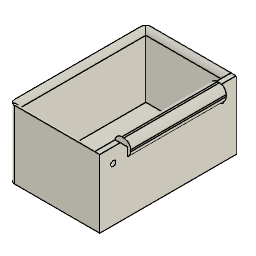
Caja Receptora Lateral (Autodesk Fusion 360 design; units mm, degrees)
Autodesk Fusion 360 part; units mm, degrees
sketch "Boceto1" plane through (0, 0, 0) normal (1, 0, 0) x (0, 1, 0)
  line L0 (0, 0) -> (80, 0)
  line L1 (80, 0) -> (80, 40)
  line L2 (80, 40) -> (0, 40)
  line L3 (0, 40) -> (0, 0)
  line L4 (80, 40) -> (80, 33)
  line L5 (80, 33) -> (80, 31.5)
  line L6 (80, 31.5) -> (72.1, 31.5)
  line L7 (0, 40) -> (0, 38.7984)
  line L8 (0, 40) -> (0, 33)
  line L9 (0, 33) -> (0, 31.5)
  line L10 (0, 31.5) -> (7.9, 31.5)
  circle A0 centre (7.9, 31.5) radius 1.525
  circle A1 centre (72.1, 31.5) radius 1.525
  dimension "d1" = 80
  dimension "d2" = 40
  dimension "d3" = 7
  dimension "d4" = 1.5
  dimension "d5" = 7.9
  dimension "d6" = 7
  dimension "d7" = 1.5
  dimension "d8" = 7.9
  dimension "d9" = 3.05
  dimension "d10" = 3.05
  constraint horizontal L0
  constraint vertical L1
  constraint horizontal L2
  constraint vertical L3
  constraint coincident L0.start L3.end
  constraint perpendicular L2 L4
  constraint perpendicular L2 L5
  constraint perpendicular L1 L6
  constraint coincident L3 L7.end
  constraint perpendicular L2 L8
  constraint perpendicular L2 L9
  constraint perpendicular L3 L10
  constraint coincident L10.end A0.centre
  constraint coincident L6.end A1.centre
  measures "d1" distance of L0.start L0.end
  measures "d2" distance of L0.start L2.end
  measures "d3" distance of L1.end L4.end
  measures "d4" distance of L4.end L5.end
  measures "d5" distance of L5.end L6.end
  measures "d6" distance of L2.end L8.end
  measures "d7" distance of L8.end L9.end
  measures "d8" distance of L9.end L10.end
  measures "d9" diameter of A0
  measures "d10" diameter of A1
extrude "Extruir1" add sketch "Boceto1" against normal blind 2 makes body 1
sketch "Boceto2" plane through (-2, 0, 0) normal (-1, 0, 0) x (0, -1, 0)
  circle A0 centre (-7.9, 31.5) radius 1.525
  circle A1 centre (-72.1, 31.5) radius 1.525
  line L0 (0, 40) -> (-80, 40)
  line L1 (-80, 40) -> (-80, 0)
  line L2 (-80, 0) -> (0, 0)
  line L3 (0, 0) -> (0, 40)
extrude "Extruir2" add sketch "Boceto2" along normal blind 1 contours A0 | A1 | L0 L1 L2 L3 bodies 1
sketch "Boceto3" plane through (0, 0, 40) normal (0, 0, 1) x (-1, 0, 0)
  line L0 (0, 0) -> (0, -80)
  line L1 (0, -80) -> (3, -80)
  line L2 (3, -80) -> (3, 0)
  line L3 (3, 0) -> (0, 0)
  line L4 (3, -80) -> (53, -80)
  line L5 (53, -80) -> (53, 0)
  line L6 (53, 0) -> (3, 0)
  line L7 (3, 0) -> (3, -80)
  line L8 (50, -3) -> (6, -3)
  line L9 (6, -3) -> (6, -77)
  line L10 (6, -77) -> (50, -77)
  line L11 (50, -77) -> (50, -3)
  line L12 (6, -77) -> (3, -77)
  line L13 (6, -3) -> (3, -3)
  dimension "d15" = 50
  dimension "d16" = -3
  constraint horizontal L4
  constraint vertical L5
  constraint horizontal L6
  constraint vertical L7
  constraint coincident L1.end L2.start
  constraint coincident L7 L12.end
  constraint perpendicular L7 L12
  constraint coincident L7 L13.end
  constraint perpendicular L7 L13
  constraint coincident L2.end L3.start
  measures "d15" distance of L1.end L4.end
extrude "Extruir3" add sketch "Boceto3" against normal up to surface (40 mm away) contours L2 L4 L5 L6 L7 L8 L10 L11 L12 L13 bodies 1
sketch "Boceto4" plane through (0, 0, 0) normal (0, 0, -1) x (1, 0, 0)
  line L0 (-3, -3) -> (-3, -77)
  line L1 (-3, -77) -> (-50, -77)
  line L2 (-50, -77) -> (-50, -3)
  line L3 (-50, -3) -> (-3, -3)
  line L4 (0, 0) -> (-53, 0)
  line L5 (-53, 0) -> (-53, -80)
  line L6 (-53, -80) -> (0, -80)
  line L7 (0, -80) -> (0, 0)
extrude "Extruir4" add sketch "Boceto4" against normal blind 3 contours L0 L1 L2 L3 bodies 1
copy_body "Cuerpo - > Comp.1" bodies 1 removing the originals makes body 2 in component "Caja Receptora"
sketch "Boceto5" plane through (0, 0, 0) normal (0, -1, 0) x (1, 0, 0)
  line L0 (0, 0) -> (0, 40)
  line L1 (0, 40) -> (-53, 40)
  line L2 (-53, 40) -> (-53, 0)
  line L3 (-53, 0) -> (0, 0)
  line L4 (0, 40) -> (-3, 40)
  line L5 (-3, 40) -> (-3, 43.5)
  line L6 (-3, 43.5) -> (0, 43.5)
  line L7 (0, 43.5) -> (0, 40)
  line L8 (0, 43.5) -> (4.15, 43.5)
  line L9 (4.15, 43.5) -> (4.15, 40)
  line L10 (4.15, 40) -> (0, 40)
  line L11 (0, 40) -> (0, 43.5)
  line L12 (4.15, 43.5) -> (6.15, 43.5)
  line L13 (6.15, 43.5) -> (6.15, 40)
  line L14 (6.15, 40) -> (4.15, 40)
  line L15 (4.15, 40) -> (4.15, 43.5)
  line L16 (4.15, 40) -> (6.15, 40)
  line L17 (6.15, 40) -> (6.15, 35)
  line L18 (6.15, 35) -> (4.15, 35)
  line L19 (4.15, 35) -> (4.15, 40)
  dimension "d21" = 3
  dimension "d22" = 3.5
  dimension "d23" = 4.15
  dimension "d24" = 3.5
  dimension "d25" = 2
  dimension "d26" = 2
  dimension "d27" = 5
  constraint horizontal L4
  constraint vertical L5
  constraint horizontal L6
  constraint vertical L7
  constraint coincident L0.end L1.start
  constraint horizontal L8
  constraint vertical L9
  constraint horizontal L10
  constraint vertical L11
  constraint horizontal L12
  constraint vertical L13
  constraint horizontal L14
  constraint vertical L15
  constraint horizontal L16
  constraint vertical L17
  constraint horizontal L18
  constraint vertical L19
  measures "d21" distance of L0.end L4.end
  measures "d22" distance of L0.end L6.end
  measures "d23" distance of L6.end L8.end
  measures "d24" distance of L6.end L0.end
  measures "d25" distance of L8.end L12.end
  measures "d26" distance of L9.end L13.end
  measures "d27" distance of L9.end L18.end
extrude "Extruir1'" add sketch "Boceto5" against normal up to surface (80 mm away) contours L1 L4 L5 L6 L7 L11 | L7 L8 L9 L10 L11 L15 | L9 L12 L13 L14 L15 L16 | L14 L16 L17 L18 L19 bodies 2 in component "Caja Receptora"
fillet "Empalme1" radius 4 3 edges at (6.15, 40, 35) (6.15, 40, 43.5) (-3, 40, 43.5) on bodies 2 in component "Caja Receptora"
fillet "Empalme2" radius 3 2 edges at (-53, 0, 20) (-53, 80, 20) on bodies 2 in component "Caja Receptora"
fillet "Empalme6" radius 3 3 edges at (-26.4843, 77, 40) (-50, 40, 40) (-26.4843, 3, 40) on bodies 2 in component "Caja Receptora"
extrude "Extruir2'" cut 2 faces at (-2, 8.2293, 31.0484) (-2, 71.3812, 31.764) along direction (-1, 0, 0) blind 1 on bodies 2 bodies 2 in component "Caja Receptora"
sketch "Boceto6" plane through (0, 80, 0) normal (0, 1, 0) x (-1, 0, 0)
  line L0 (50, 0) -> (50, 40)
  line L1 (50, 40) -> (2.9686, 40)
  arc A0 (2.9686, 40) -> (-1, 43.5) centre (-1, 39.5) ccw
  line L2 (-1, 43.5) -> (-2.15, 43.5)
  arc A1 (-2.15, 43.5) -> (-6.15, 39.5) centre (-2.15, 39.5) ccw
  line L3 (-6.15, 39.5) -> (-6.15, 38.4641)
  arc A2 (-6.15, 38.4641) -> (-4.15, 35) centre (-2.15, 38.4641) ccw
  line L4 (-4.15, 35) -> (-4.15, 40)
  line L5 (-4.15, 40) -> (0, 40)
  line L6 (0, 40) -> (0, 0)
  line L7 (0, 0) -> (50, 0)
  line L8 (2.9686, 40) -> (0, 40)
  constraint coincident L1.end A0.start
  constraint coincident L5.end L6.start
extrude "Extruir3'" cut sketch "Boceto6" against normal blind 12 contours A0 L2 A1 L3 A2 L4 L5 L8 bodies 2 in component "Caja Receptora"
sketch "Boceto7" plane through (0, 0, 0) normal (0, -1, 0) x (1, 0, 0)
  line L0 (-50, 40) -> (-50, 0)
  line L1 (-50, 0) -> (0, 0)
  line L2 (0, 0) -> (0, 40)
  line L3 (0, 40) -> (4.15, 40)
  line L4 (4.15, 40) -> (4.15, 35)
  arc A0 (4.15, 35) -> (6.15, 38.4641) centre (2.15, 38.4641) ccw
  line L5 (6.15, 38.4641) -> (6.15, 39.5)
  arc A1 (6.15, 39.5) -> (2.15, 43.5) centre (2.15, 39.5) ccw
  line L6 (2.15, 43.5) -> (1, 43.5)
  arc A2 (1, 43.5) -> (-2.9686, 40) centre (1, 39.5) ccw
  line L7 (-2.9686, 40) -> (-50, 40)
  line L8 (0, 40) -> (-2.9686, 40)
  constraint coincident L2.end L3.start
  constraint coincident A2.end L7.start
extrude "Extruir4'" cut sketch "Boceto7" against normal blind 12 contours L3 L4 A0 L5 A1 L6 A2 L8 bodies 2 in component "Caja Receptora"
component "Caja Receptora" placed x (1, 0, 0) y (0, 1, 0) z (0, 0, 1) at (0, 0, 0)
named bodies: "Caja Receptora"
